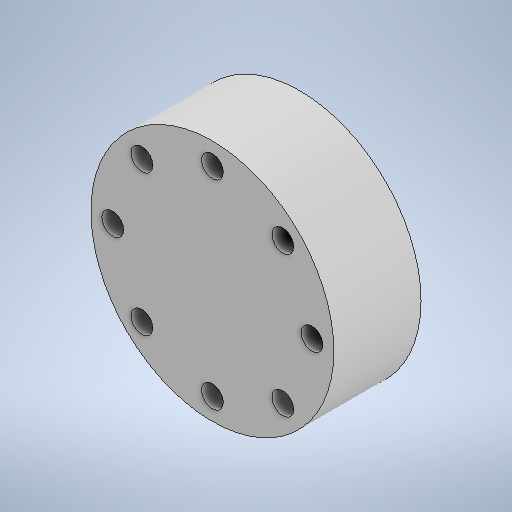
# Autodesk Inventor part: horn_3
Saved by Autodesk Inventor 2025.2 (Build 292293000, 293)
## iProperties
Created: 2025-02-13
Part Number: horn_3
Material: Generic
Document SubType Name: Modeling
Designer: Admin
Density: 1 g/cm^3
Appearance: Default
Author: Admin
Autodesk Inventor part; units mm, degrees
ref_plane "YZ Plane" through (0, 0, 0) normal (1, 0, 0) x (0, 1, 0)
ref_plane "XZ Plane" through (0, 0, 0) normal (0, 1, 0) x (-1, 0, 0)
ref_plane "XY Plane" through (0, 0, 0) normal (0, 0, 1) x (1, 0, 0)
sketch "Sketch2" plane through (0, 0, 0) normal (0, 0, 1) x (1, 0, 0)
  circle A0 centre (0, 8) radius 0.875
  circle A1 centre (0, 0) radius 1
  circle A2 centre (-5.6569, 5.6569) radius 0.875
  circle A3 centre (-8, 0) radius 0.875
  circle A4 centre (-5.6569, -5.6569) radius 0.875
  circle A5 centre (0, -8) radius 0.875
  circle A6 centre (5.6569, -5.6569) radius 0.875
  circle A7 centre (8, 0) radius 0.875
  circle A8 centre (5.6569, 5.6569) radius 0.875
  circle A9 centre (0, 0) radius 9.75
  circle A10 centre (0, 0) radius 4
  point P0 (0.1028, -10.875)
  dimension "d5" = 360
  dimension "d10" = 1.75
  dimension "d11" = 19.5
  dimension "d12" = 8
  dimension "d13" = 2
  constraints: 11 centre point, 3 coincident, 17 other
  measures "d10" diameter of A7
  measures "d11" diameter of A9
  measures "d12" diameter of A10
  measures "d13" diameter of A1
extrude "Extrusion1" add sketch "Sketch2" along normal blind 5 contours A9
sketch "Sketch4" plane through (0, 0, 5) normal (0, 0, 1) x (1, 0, 0)
  circle A0 centre (0, 0) radius 9.75 projected
  circle A1 centre (0, 0) radius 4 projected
  circle A2 centre (5.6569, 5.6569) radius 0.875 projected
  circle A3 centre (8, 0) radius 0.875 projected
  circle A4 centre (5.6569, -5.6569) radius 0.875 projected
  circle A5 centre (0, -8) radius 0.875 projected
  circle A6 centre (-5.6569, -5.6569) radius 0.875 projected
  circle A7 centre (-8, 0) radius 0.875 projected
  circle A8 centre (-5.6569, 5.6569) radius 0.875 projected
  circle A9 centre (0, 8) radius 0.875 projected
extrude "Extrusion3" add sketch "Sketch4" along normal blind 2 contours A0 | A1
body "Solid1"
